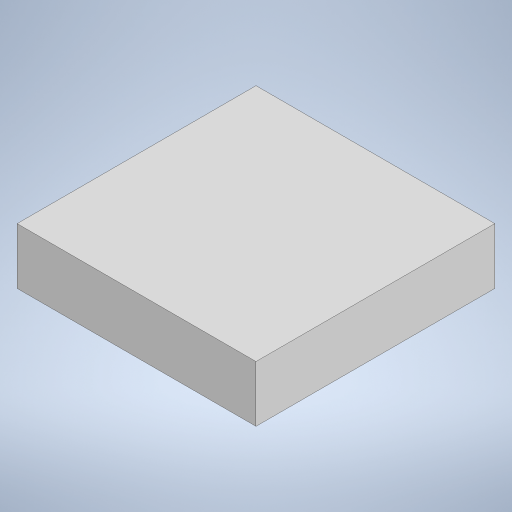
# Autodesk Inventor part: OV-PAM_n_4_standard_1F
Saved by Autodesk Inventor 2024 (Build 280153000, 153)
## iProperties
Created: 2023-08-31
Part Number: OV-PAM_n_4_standard_1F
Material: 일반
Document SubType Name: Modeling
Designer: jsw
Density: 1 g/cm^3
Appearance: 기본값
Author: jsw
Autodesk Inventor part; units mm, degrees
ref_plane "YZ Plane" through (0, 0, 0) normal (1, 0, 0) x (0, 1, 0)
ref_plane "XZ Plane" through (0, 0, 0) normal (0, 1, 0) x (-1, 0, 0)
ref_plane "XY Plane" through (0, 0, 0) normal (0, 0, 1) x (1, 0, 0)
sketch "스케치1" plane through (0, 0, 0) normal (0, 1, 0) x (-1, 0, 0)
  line L0 (-24.9446, 24.9446) -> (24.9446, 24.9446)
  line L1 (24.9446, 24.9446) -> (24.9446, -24.9446)
  line L2 (24.9446, -24.9446) -> (-24.9446, -24.9446)
  line L3 (-24.9446, -24.9446) -> (-24.9446, 24.9446)
  line L4 (-24.9446, 24.9446) -> (24.9446, -24.9446) construction
  line L5 (24.9446, 24.9446) -> (-24.9446, -24.9446) construction
  line L6 (-25.5446, 25.5446) -> (25.5446, 25.5446)
  line L7 (25.5446, 25.5446) -> (25.5446, -25.5446)
  line L8 (25.5446, -25.5446) -> (-25.5446, -25.5446)
  line L9 (-25.5446, -25.5446) -> (-25.5446, 25.5446)
  line L10 (-25.5446, 25.5446) -> (25.5446, -25.5446) construction
  line L11 (25.5446, 25.5446) -> (-25.5446, -25.5446) construction
  point P0 (0, 0)
  dimension "d0" = 70.554
  dimension "d1" = 0.6
  constraints: 24 end point, 4 midpoint, 4 parallel, 4 perpendicular, 2 horizontal
  measures "d0" distance of L0.start L1.end
  measures "d1" distance between parallel lines of L1 L7
extrude "돌출1" add sketch "스케치1" along normal blind 12 contours L0 L1 L2 L3 | L6 L7 L8 L9
